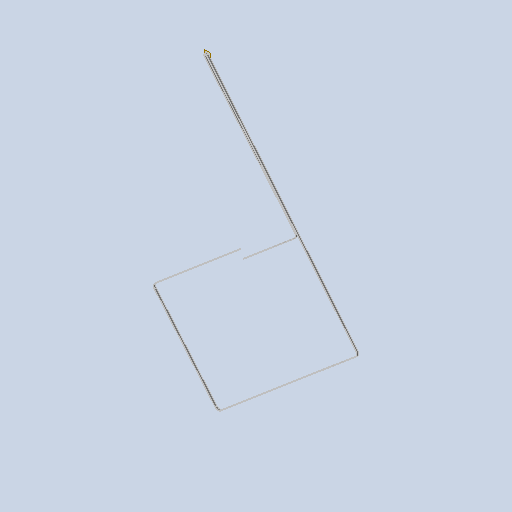
# Autodesk Inventor part: Belt1
Saved by Autodesk Inventor 2023 (Build 270158000, 158)
## iProperties
Created: 2023-08-16
Part Number: Belt1
Material: Generic
Document SubType Name: Modeling
Designer: Felix
Density: 1 g/cm^3
Appearance: Smooth - Black
Author: Felix
Autodesk Inventor part; units mm, degrees
ref_plane "YZ Plane" through (0, 0, 0) normal (1, 0, 0) x (0, 1, 0)
ref_plane "XZ Plane" through (0, 0, 0) normal (0, 1, 0) x (-1, 0, 0)
ref_plane "Work Plane1" through (0, 0, 0.5) normal (0, 0, 1) x (1, 0, 0)
sketch "Sketch1" plane through (0, 0, 0.5) normal (0, 0, 1) x (1, 0, 0)
  arc A0 (4.1391, 2.5087) -> (3.9017, 2.864) centre (0, 0) ccw construction
  arc A1 (1.2602, 4.4787) -> (2.2758, 4.058) centre (1.7603, 4.2498) ccw construction
  circle A2 centre (0, 0) radius 4.05 construction
  circle A3 centre (284.3339, -363.0367) radius 11 construction
  circle A4 centre (483.573, -598.8165) radius 11 construction
  circle A5 centre (41.6311, -972.2671) radius 11 construction
  circle A6 centre (-157.608, -736.4873) radius 11 construction
  line L0 (110.2354, -491.8247) -> (106.3399, -495.1165) construction
  line L1 (108.2876, -493.4706) -> (162.0638, -557.1094) construction
  line L2 (110.2239, -495.762) -> (-164.7078, -728.0854)
  line L3 (-166.0099, -743.5871) -> (33.2292, -979.3669)
  line L4 (48.7309, -980.669) -> (490.6728, -607.2184)
  line L5 (492.0682, -591.8285) -> (3.1278, 2.5728)
  arc A7 (3.1278, 2.5728) -> (-3.0968, -2.6101) centre (0, 0) ccw
  arc A8 (-164.7078, -728.0854) -> (-166.0099, -743.5871) centre (-157.608, -736.4873) ccw
  arc A9 (33.2292, -979.3669) -> (48.7309, -980.669) centre (41.6311, -972.2671) ccw
  arc A10 (490.6728, -607.2184) -> (492.0682, -591.8285) centre (483.573, -598.8165) ccw
  circle A11 centre (284.3339, -363.0367) radius 12.5 construction
  line L6 (292.4019, -372.5844) -> (125.3917, -513.7116)
  line L7 (-3.0968, -2.6101) -> (293.8919, -354.981)
  arc A12 (292.4019, -372.5844) -> (293.8919, -354.981) centre (284.3339, -363.0367) ccw
  line L8 (124.4236, -512.5659) -> (291.4337, -371.4387)
  arc A13 (291.4337, -371.4387) -> (292.7449, -355.9477) centre (284.3339, -363.0367) ccw
  line L9 (292.7449, -355.9477) -> (-4.2437, -3.5768)
  arc A14 (4.2862, 3.5257) -> (-4.2437, -3.5768) centre (0, 0) ccw
  line L10 (4.2862, 3.5257) -> (493.2266, -590.8756)
  arc A15 (491.641, -608.3641) -> (493.2266, -590.8756) centre (483.573, -598.8165) ccw
  line L11 (491.641, -608.3641) -> (49.6991, -981.8147)
  arc A16 (32.0835, -980.335) -> (49.6991, -981.8147) centre (41.6311, -972.2671) ccw
  line L12 (32.0835, -980.335) -> (-167.1556, -744.5553)
  arc A17 (-165.6759, -726.9396) -> (-167.1556, -744.5553) centre (-157.608, -736.4873) ccw
  line L13 (-165.6759, -726.9396) -> (109.2558, -494.6163)
  line L14 (125.3917, -513.7116) -> (124.4236, -512.5659)
  line L15 (109.2558, -494.6163) -> (110.2239, -495.762)
  point P0 (0, 0)
extrude "Extrusion1" add sketch "Sketch1" along normal blind 6
equation "\"d2\" = d1"
equation "\"d1\" = 1.5"
body "Solid1"
